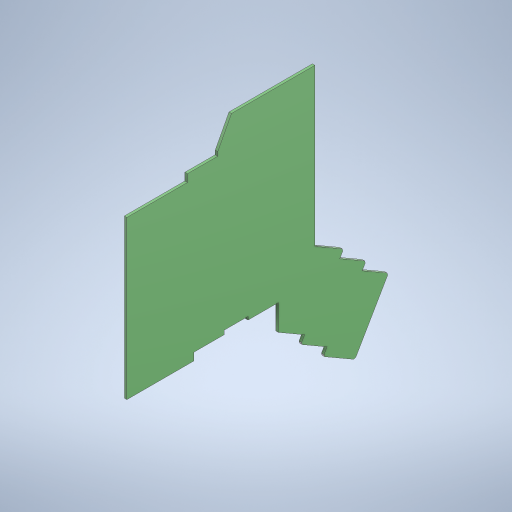
# Autodesk Inventor part: board-profile
Saved by Autodesk Inventor 2024.1 (Build 281209000, 209)
## iProperties
Created: 2023-11-07
Part Number: board-profile
Material: Générique
Document SubType Name: Modeling
Designer: Thibault
Density: 1 g/cm^3
Appearance: Par défaut
Author: Thibault
Autodesk Inventor part; units mm, degrees
ref_plane "YZ Plane" through (0, 0, 0) normal (1, 0, 0) x (0, 1, 0)
ref_plane "XZ Plane" through (0, 0, 0) normal (0, 1, 0) x (-1, 0, 0)
ref_plane "XY Plane" through (0, 0, 0) normal (0, 0, 1) x (1, 0, 0)
sketch "Key" plane through (0, 0, 0) normal (0, 0, 1) x (1, 0, 0)
  line L0 (-9.525, 9.525) -> (9.525, 9.525) construction
  line L1 (9.525, 9.525) -> (9.525, -9.525) construction
  line L2 (9.525, -9.525) -> (-9.525, -9.525) construction
  line L3 (-9.525, -9.525) -> (-9.525, 9.525) construction
  line L4 (-9.525, 9.525) -> (9.525, -9.525) construction
  line L5 (9.525, 9.525) -> (-9.525, -9.525) construction
  point P0 (0, 0)
  point P1 (0, 0)
  dimension "d6" = 19.05
  dimension "d7" = 19.05
  measures "d6" distance of L1.end L2.end
  measures "d7" distance of L0.end L1.end
sketch "Col5" plane through (0, 0, 0) normal (0, 0, 1) x (1, 0, 0)
  point P0 (-10.8651, 0)
sketch "Col4" plane through (0, 0, 0) normal (0, 0, 1) x (1, 0, 0)
  point P0 (-10.8651, 0)
sketch "TC" plane through (0, 0, 0) normal (0, 0, 1) x (1, 0, 0)
  point P0 (-22.1335, 152.0917)
  dimension "d12" = 4.7625
  dimension "d13" = 4.7625
  dimension "d14" = 19.6363
sketch "Esquisse1" plane through (0, 0, 0) normal (1, 0, 0) x (0, 1, 0)
  line L0 (28.177, -71.755) -> (10.397, -71.755) construction
  line L1 (10.397, -71.755) -> (10.397, -102.235) construction
  line L2 (10.397, -102.235) -> (28.177, -102.235)
  line L3 (28.177, -102.235) -> (28.177, -71.755) construction
  line L4 (28.177, -71.755) -> (10.397, -102.235) construction
  line L5 (10.397, -71.755) -> (28.177, -102.235) construction
  line L6 (6.445, 14.065) -> (-92.805, 14.065)
  line L7 (6.445, 14.065) -> (6.445, -24.035)
  line L8 (-68.4861, -104.235) -> (30.177, -104.235)
  line L9 (30.177, -51.755) -> (30.177, -104.235)
  line L10 (-106.1694, -150.4545) -> (-142.6291, -129.4045)
  line L11 (-103.8052, -81.2096) -> (-113.3302, -97.7073)
  line L12 (-113.3302, -97.7073) -> (-117.4547, -95.3261)
  line L13 (-117.4547, -95.3261) -> (-126.9797, -111.8239)
  line L14 (-126.9797, -111.8239) -> (-131.1041, -109.4426)
  line L15 (-131.1041, -109.4426) -> (-142.6291, -129.4045)
  line L16 (-68.4861, -104.235) -> (-78.8706, -122.2214)
  line L17 (-78.8706, -122.2214) -> (-82.995, -119.8402)
  line L18 (-82.995, -119.8402) -> (-92.52, -136.338)
  line L19 (-92.52, -136.338) -> (-96.6444, -133.9567)
  line L20 (-96.6444, -133.9567) -> (-106.1694, -150.4545)
  line L21 (-92.805, 14.065) -> (-92.805, -28.035)
  line L22 (-92.805, -28.035) -> (-88.042, -28.035)
  line L23 (-88.042, -28.035) -> (-88.042, -47.085)
  line L24 (-88.042, -47.085) -> (-85.565, -47.085)
  line L25 (-85.565, -47.085) -> (-85.565, -62.135)
  line L26 (-85.565, -62.135) -> (-87.565, -62.135)
  line L27 (-89.5164, -89.4592) -> (-103.8052, -81.2096) construction
  line L28 (6.445, -24.035) -> (11.208, -24.035)
  line L29 (11.208, -24.035) -> (11.208, -43.085)
  line L30 (11.208, -43.085) -> (13.685, -43.085)
  line L31 (30.177, -51.755) -> (13.685, -43.085)
  line L32 (-78.8706, -122.2214) -> (-92.52, -136.338) construction
  line L33 (-92.52, -136.338) -> (-106.1694, -150.4545) construction
  line L34 (-103.8052, -81.2096) -> (-117.4547, -95.3261) construction
  line L35 (-131.1041, -109.4426) -> (-117.4547, -95.3261) construction
  line L36 (-103.8052, -81.2096) -> (-87.565, -81.2096)
  line L37 (-87.565, -81.2096) -> (-87.565, -62.135)
  point P0 (-5.08, 2.54)
  point P1 (19.287, -86.995)
  point P2 (-5.08, 2.54)
  point P3 (-86.042, -35.56)
  point P4 (0, 0)
extrude "Extrusion1" add sketch "Esquisse1" along normal blind 1.6
chamfer "Chanfrein5" distance 1 angle 45 6 edges at (0.8, -117.4547, -95.3261) (0.8, -131.1041, -109.4426) (0.8, -142.6291, -129.4045) (0.8, -106.1694, -150.4545) (0.8, -92.52, -136.338) (0.8, -78.8706, -122.2214)
